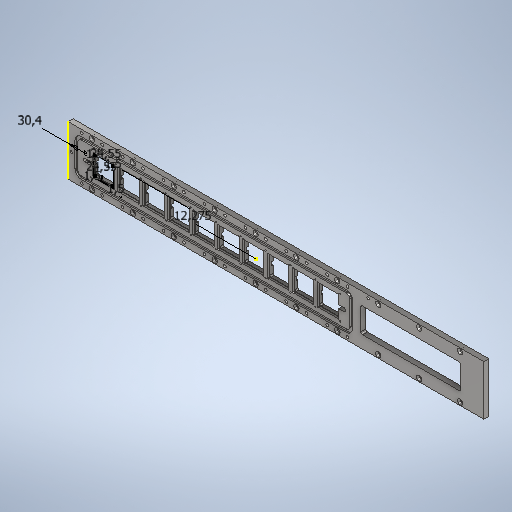
# Autodesk Inventor part: Bauteil6
Saved by Autodesk Inventor 2025.2 (Build 292293000, 293)
## iProperties
Created: 2024-12-16
Part Number: Bauteil6
Material: Edelstahl
Document SubType Name: Modeling
Designer: gorenfl4
Density: 8 g/cm^3
Appearance: Halbpoliert
Mass: 624.845 g
Surface Area: 428.772 cm^2
Volume: 78.1056 cm^3
Author: gorenfl4
Autodesk Inventor part; units mm, degrees
ref_plane "YZ Plane" through (0, 0, 0) normal (1, 0, 0) x (0, 1, 0)
ref_plane "XZ Plane" through (0, 0, 0) normal (0, 1, 0) x (-1, 0, 0)
ref_plane "XY Plane" through (0, 0, 0) normal (0, 0, 1) x (1, 0, 0)
sketch "Skizze1" plane through (0, 0, 0) normal (0, 1, 0) x (-1, 0, 0)
  line L0 (226, 30) -> (-274, 30)
  line L1 (-274, 30) -> (-274, -30)
  line L2 (-274, -30) -> (226, -30)
  line L3 (226, -30) -> (226, 30)
  point P0 (0, 0)
  dimension "d0" = 274
  dimension "d1" = 500
  dimension "d2" = 60
  dimension "d3" = 30
  constraints: 8 end point, 2 parallel, 1 horizontal, 1 perpendicular
  measures "d0" distance from line of point (0, 0) L1
  measures "d1" distance between parallel lines of L1 L3
  measures "d2" distance between parallel lines of L2 L0
  measures "d3" distance from line of point (0, 0) L2
extrude "Extrusion1" add sketch "Skizze1" along normal blind 6
sketch "Skizze4" plane through (0, 0, 0) normal (0, -1, 0) x (1, 0, 0)
  line L0 (-195.6, -10.775) -> (-195.6, 10.775)
  line L1 (-226, -30) -> (-226, 30) projected
  arc A0 (-194.1, 12.275) -> (-195.6, 10.775) centre (-194.1, 10.775) ccw
  arc A1 (-195.6, -10.775) -> (-194.1, -12.275) centre (-194.1, -10.775) ccw
  line L2 (-194.1, 12.275) -> (-172.55, 12.275)
  line L3 (-194.1, -12.275) -> (-172.55, -12.275)
  arc A2 (-172.55, -12.275) -> (-171.05, -10.775) centre (-172.55, -10.775) ccw
  arc A3 (-171.05, 10.775) -> (-172.55, 12.275) centre (-172.55, 10.775) ccw
  line L4 (-171.05, 10.775) -> (-171.05, -10.775)
  point P0 (0, 0)
  point P1 (-193.6, -12)
  dimension "d29" = 30.4
  dimension "d35" = 24.55
  dimension "d36" = 24.55
  dimension "d298" = 12.275
  dimension "d299" = 1.5
  dimension "d300" = 1.5
  dimension "d301" = 1.5
  dimension "d302" = 1.5
  constraints: 8 end point, 8 point on circle, 8 tangent, 4 centre point, 2 horizontal, 2 vertical
  measures "d29" distance between parallel lines of L1 L0
  measures "d35" distance between parallel lines of L4 L0
  measures "d36" distance between parallel lines of L2 L3
  measures "d298" distance from line of point (0, 0) L2
  measures "d299" radius of A1
  measures "d300" radius of A2
  measures "d301" radius of A3
  measures "d302" radius of A0
extrude "Extrusion3" cut sketch "Skizze4" against normal through all
pattern_linear "Rechteckige Anordnung2" count 10 spacing 30 along (1, 0, 0) of "Extrusion3"
sketch "Skizze18" plane through (0, 0, 0) normal (0, -1, 0) x (1, 0, 0)
  line L0 (98.95, -10.775) -> (98.95, 10.775) projected
  line L1 (98.95, -2) -> (105.95, -2)
  line L2 (105.95, 2) -> (98.95, 2)
  line L3 (98.95, 2) -> (98.95, -2)
  arc A0 (105.95, -2) -> (105.95, 2) centre (105.95, 0) ccw
  point P0 (0, 0)
  point P1 (64.65, 0)
  dimension "d154" = 2
  dimension "d155" = 2
  dimension "d159" = 7
  dimension "d160" = 2
  constraints: 6 end point, 2 point on circle, 1 centre point, 1 horizontal, 1 parallel, 1 point on line, 1 tangent
  measures "d154" distance from line of L1 point (64.65, 0)
  measures "d155" distance from line of L2 point (64.65, 0)
  measures "d159" distance from line of A0.centre L0
  measures "d160" radius of A0
extrude "Extrusion6" cut sketch "Skizze18" against normal through all
sketch "Skizze19" plane through (0, 0, 0) normal (0, -1, 0) x (1, 0, 0)
  line L0 (-210.35, -18.775) -> (108.45, -18.775)
  line L1 (108.45, 18.775) -> (-210.35, 18.775)
  circle A0 centre (-219.85, 14.5) radius 0.7835 projected
  arc A1 (-210.35, 18.775) -> (-214.35, 14.775) centre (-210.35, 14.775) ccw
  arc A2 (108.45, -18.775) -> (112.45, -14.775) centre (108.45, -14.775) ccw
  arc A3 (112.45, 14.775) -> (108.45, 18.775) centre (108.45, 14.775) ccw
  line L2 (112.45, -14.775) -> (112.45, 14.775)
  arc A4 (-214.35, -14.775) -> (-210.35, -18.775) centre (-210.35, -14.775) ccw
  line L3 (-214.35, -14.775) -> (-214.35, 14.775)
  line L4 (108.45, -22.325) -> (-210.35, -22.325)
  arc A5 (-217.9, -14.775) -> (-210.35, -22.325) centre (-210.35, -14.775) ccw
  line L5 (-217.9, -14.775) -> (-217.9, 14.775)
  arc A6 (-210.35, 22.325) -> (-217.9, 14.775) centre (-210.35, 14.775) ccw
  line L6 (-210.35, 22.325) -> (108.45, 22.325)
  arc A7 (116, 14.775) -> (108.45, 22.325) centre (108.45, 14.775) ccw
  line L7 (116, 14.775) -> (116, -14.775)
  arc A8 (108.45, -22.325) -> (116, -14.775) centre (108.45, -14.775) ccw
  line L8 (-194.1, 12.275) -> (-172.55, 12.275) projected
  line L9 (-172.55, -12.275) -> (-194.1, -12.275) projected
  arc A9 (105.95, -2) -> (105.95, 2) centre (105.95, 0) ccw projected
  line L10 (-195.6, -10.775) -> (-195.6, 10.775) projected
  line L11 (-226, -30) -> (-226, 30) projected
  point P0 (0, 0)
  dimension "d166" = 4
  dimension "d167" = 4
  dimension "d168" = 3.55
  dimension "d242" = 6.5
  dimension "d243" = 6.5
  dimension "d244" = 6.5
  dimension "d252" = 8.1
  dimension "d253" = 4
  dimension "d254" = 4
  constraints: 17 end point, 16 point on circle, 8 centre point, 8 tangent, 2 parallel, 2 vertical, 1 horizontal, 7 other
  measures "d166" radius of A2
  measures "d167" radius of A3
  measures "d168" distance between parallel lines of L0 L4
  measures "d242" distance between parallel lines of L8 L1
  measures "d243" distance between parallel lines of L0 L9
  measures "d244" distance from line of A9.centre L2
  measures "d252" distance between parallel lines of L11 L5
  measures "d253" radius of A4
  measures "d254" radius of A1
extrude "Extrusion7" cut sketch "Skizze19" against normal blind 1.9 contours L4 A5 L5 A6 L6 A7 L7 A8
sketch "Skizze21" plane through (0, 0, 0) normal (0, -1, 0) x (1, 0, 0)
  line L0 (274, -30) -> (-226, -30) projected
  line L1 (-226, -30) -> (-226, 30) projected
  point P0 (0, 0)
  point P1 (-222.25, 0)
  dimension "d180" = 30
  dimension "d181" = 3.75
  measures "d180" distance from line of L0 point (-222.25, 0)
  measures "d181" distance from line of L1 point (-222.25, 0)
hole "Bohrung12" at (-222.25, 0, 0) direction (0, 1, 0) diameter 3 end through all
sketch "Skizze26" plane through (0, 0, 0) normal (0, -1, 0) x (1, 0, 0)
  line L0 (-195.6, -10.775) -> (-195.6, 10.775) projected
  line L1 (-195.6, -2) -> (-206.1, -2)
  line L2 (-195.6, 2) -> (-206.1, 2)
  arc A0 (-206.1, 2) -> (-206.1, -2) centre (-206.1, 0) ccw
  point P0 (0, 0)
  dimension "d246" = 4
  dimension "d247" = 2
  dimension "d248" = 10.5
  constraints: 4 end point, 2 horizontal, 2 point on circle, 2 point on line, 1 centre point, 1 tangent
  measures "d246" distance between parallel lines of L1 L2
  measures "d247" radius of A0
  measures "d248" distance from line of L0 A0.centre
extrude "Extrusion9" cut sketch "Skizze26" against normal through all
sketch "Skizze27" plane through (0, 0, 0) normal (0, -1, 0) x (1, 0, 0)
  line L0 (-195.6, 2) -> (-195.6, 10.775) projected
  line L1 (-194.1, 12.275) -> (-172.55, 12.275) projected
  point P0 (0, 0)
  point P1 (-198.6, 14.275)
  dimension "d255" = 3
  dimension "d256" = 2
  measures "d255" distance from line of L0 point (-198.6, 14.275)
  measures "d256" distance from line of L1 point (-198.6, 14.275)
hole "Bohrung15" at (-198.6, 0, 14.275) direction (0, 1, 0) diameter 1.567 end through all thread size "M2x0.4" class "6H" standard "ISO Metric profile"
sketch "Skizze28" plane through (0, 0, 0) normal (0, -1, 0) x (1, 0, 0)
  line L0 (-195.6, -10.775) -> (-195.6, -2) projected
  line L1 (-172.55, -12.275) -> (-194.1, -12.275) projected
  point P0 (0, 0)
  point P1 (-198.6, -14.275)
  dimension "d264" = 3
  dimension "d265" = 2
  measures "d264" distance from line of L0 point (-198.6, -14.275)
  measures "d265" distance from line of L1 point (-198.6, -14.275)
hole "Bohrung16" at (-198.6, 0, -14.275) direction (0, 1, 0) diameter 1.567 end through all thread size "M2x0.4" class "6H" standard "ISO Metric profile"
pattern_linear "Rechteckige Anordnung7" count 11 spacing 30 along (1, 0, 0) of "Bohrung15", "Bohrung16"
sketch "Skizze33" plane through (0, 0, 0) normal (0, -1, 0) x (1, 0, 0)
  line L0 (-194.65, 12.825) -> (-172, 12.825)
  line L1 (-195.6, 2) -> (-195.6, 10.775) projected
  arc A0 (-194.65, 12.825) -> (-196.15, 12.825) centre (-195.4, 12.825) ccw
  line L2 (-206.1, 2) -> (-195.6, 2) projected
  line L3 (-196.15, 12.825) -> (-196.15, -12.825)
  line L4 (-195.6, -2) -> (-195.6, -10.775) projected
  line L5 (-194.1, 12.275) -> (-172.55, 12.275) projected
  line L6 (-194.65, -12.825) -> (-172, -12.825)
  line L7 (-172.55, -12.275) -> (-194.1, -12.275) projected
  arc A1 (-196.15, -12.825) -> (-194.65, -12.825) centre (-195.4, -12.825) ccw
  line L8 (-170.5, 12.825) -> (-170.5, -12.825)
  line L9 (-171.05, 10.775) -> (-171.05, -10.775) projected
  arc A2 (-172, -12.825) -> (-170.5, -12.825) centre (-171.25, -12.825) ccw
  arc A3 (-170.5, 12.825) -> (-172, 12.825) centre (-171.25, 12.825) ccw
  point P0 (0, 0)
  dimension "d304" = 0.75
  dimension "d305" = 0.55
  dimension "d306" = 0.55
  dimension "d307" = 0.55
  dimension "d308" = 0.75
  dimension "d309" = 0.55
  dimension "d310" = 0.75
  dimension "d311" = 0.75
  constraints: 9 end point, 8 point on circle, 4 centre point, 4 line through centre, 4 tangent, 2 horizontal, 1 parallel, 1 vertical
  measures "d304" radius of A0
  measures "d305" distance between parallel lines of L0 L5
  measures "d306" distance between parallel lines of L3 L1
  measures "d307" distance between parallel lines of L6 L7
  measures "d308" radius of A1
  measures "d309" distance between parallel lines of L9 L8
  measures "d310" radius of A2
  measures "d311" radius of A3
extrude "Extrusion10" cut sketch "Skizze33" against normal blind 2.2
pattern_linear "Rechteckige Anordnung8" count 10 spacing 30 along (1, 0, 0) of "Extrusion10"
sketch "Skizze34" plane through (0, 6, 0) normal (0, 1, 0) x (1, 0, 0)
  line L0 (74.4, -10.775) -> (74.4, 10.775) projected
  line L1 (-171.05, 10.775) -> (-171.05, -10.775) projected
  line L2 (74.4, 2) -> (-171.05, 2)
  line L3 (-171.05, 2) -> (-171.05, -2)
  line L4 (-171.05, -2) -> (74.4, -2)
  line L5 (74.4, -2) -> (74.4, 2)
  point P0 (0, 0)
  point P1 (74.4, 0)
  dimension "d317" = 2
  dimension "d318" = 2
  constraints: 8 end point, 2 parallel, 2 point on line, 1 horizontal, 1 midpoint, 1 perpendicular
  measures "d317" distance from line of point (0, 0) L2
  measures "d318" distance from line of L4 point (74.4, 0)
extrude "Extrusion11" cut sketch "Skizze34" against normal blind 2.2
sketch "Skizze36" plane through (0, 0, 0) normal (0, -1, 0) x (1, 0, 0)
  line L0 (-226, -30) -> (-226, 30) projected
  line L1 (274, -30) -> (-226, -30) projected
  point P0 (0, 0)
  point P1 (-197.4, -26.25)
  dimension "d322" = 28.6
  dimension "d323" = 3.75
  measures "d322" distance from line of L0 point (-197.4, -26.25)
  measures "d323" distance from line of L1 point (-197.4, -26.25)
hole "Festschraubung Zentrierplatte" at (-197.4, 0, -26.25) direction (0, 1, 0) diameter 3.4 end through all counterbore diameter 6.5 counterbore depth 3 clearance for "Innensechskantkopfschraube" size "M3" standard "ANSI Metrisches M Profil"
pattern_linear "Rechteckige Anordnung9" count 10 spacing 49.2 along (1, 0, 0) count 2 spacing 52.5 along (0, 0, 1) of "Festschraubung Zentrierplatte"
sketch "Skizze37" plane through (0, 0, 0) normal (0, -1, 0) x (1, 0, 0)
  line L0 (-226, 30) -> (274, 30) projected
  line L1 (-226, -30) -> (-226, 30) projected
  point P0 (0, 0)
  point P1 (-209.7, 26.25)
  dimension "d337" = 3.75
  dimension "d345" = 16.3
  measures "d337" distance from line of L0 point (-209.7, 26.25)
  measures "d345" distance from line of L1 point (-209.7, 26.25)
hole "Durchgangsbohrung" at (-209.7, 0, 26.25) direction (0, 1, 0) diameter 3.4 end through all clearance for "Flachkopfmaschinenschraube" size "M3" standard "ANSI Metrisches M Profil"
pattern_linear "Durchgangsbohrungen" count 14 spacing 24.6 along (1, 0, 0) count 2 spacing 52.5 along (0, 0, -1) of "Durchgangsbohrung"
sketch "Skizze38" plane through (0, 6, 0) normal (0, 1, 0) x (1, 0, 0)
  line L0 (126, -15) -> (246, -15)
  line L1 (246, -15) -> (246, 15)
  line L2 (246, 15) -> (126, 15)
  line L3 (126, 15) -> (126, -15)
  line L4 (-226, -30) -> (274, -30) projected
  line L5 (274, 30) -> (-226, 30) projected
  line L6 (274, -30) -> (274, 30) projected
  point P0 (0, 0)
  dimension "d352" = 15
  dimension "d353" = 15
  dimension "d354" = 28
  dimension "d355" = 120
  constraints: 8 end point, 2 parallel, 1 horizontal, 1 perpendicular
  measures "d352" distance between parallel lines of L4 L0
  measures "d353" distance between parallel lines of L5 L2
  measures "d354" distance between parallel lines of L6 L1
  measures "d355" distance between parallel lines of L1 L3
extrude "Extrusion12" cut sketch "Skizze38" against normal through all
fillet "Rundung1" radius 2 4 edges at (126, 3, 15) (246, 3, 15) (246, 3, -15) (126, 3, -15)
sketch "Skizze39" plane through (0, 0, 0) normal (0, -1, 0) x (1, 0, 0)
  line L0 (-226, -30) -> (-226, 30) projected
  line L1 (-226, 30) -> (274, 30) projected
  point P0 (0, 0)
  point P1 (134.7, 26.25)
  dimension "d359" = 360.7
  dimension "d367" = 3.75
  measures "d359" distance from line of L0 point (134.7, 26.25)
  measures "d367" distance from line of L1 point (134.7, 26.25)
hole "Bohrung21" at (134.7, 0, 26.25) direction (0, 1, 0) diameter 3 end through all
